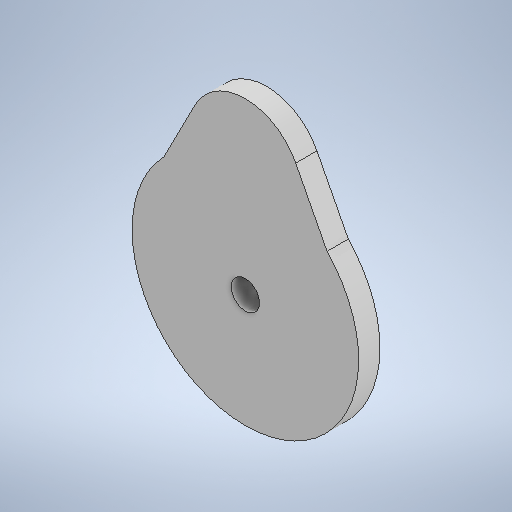
# Autodesk Inventor part: Part_Pear_Cam
Saved by Autodesk Inventor 2025 (Build 290162010, 162A)
## iProperties
Created: 2023-01-24
Part Number: Part_Pear_Cam
Material: Generic
Document SubType Name: Modeling
Designer: kani2
Density: 1 g/cm^3
Appearance: Default
Author: kani2
Autodesk Inventor part; units mm, degrees
ref_plane "YZ Plane" through (0, 0, 0) normal (1, 0, 0) x (0, 1, 0)
ref_plane "XZ Plane" through (0, 0, 0) normal (0, 1, 0) x (-1, 0, 0)
ref_plane "XY Plane" through (0, 0, 0) normal (0, 0, 1) x (1, 0, 0)
sketch "Sketch1" plane through (0, 0, 0) normal (0, 0, 1) x (1, 0, 0)
  arc A0 (-18.3123, 17.6017) -> (18.3123, 17.6017) centre (0, 0) ccw
  line L0 (-18.3123, 17.6017) -> (-11.287, 31.2218)
  line L1 (18.3123, 17.6017) -> (11.287, 31.2218)
  arc A1 (11.287, 31.2218) -> (-11.287, 31.2218) centre (0, 25.4) ccw
  dimension "d0" = 50.8
  dimension "d2" = 25.4
  constraints: 4 end point, 4 point on circle, 2 centre point, 2 tangent, 1 coincident
  measures "d0" diameter of A0
  measures "d2" distance of point (0, 0) A1.centre
extrude "Extrusion1" add sketch "Sketch1" along normal blind 4.7625
sketch "Sketch2" plane through (0, 0, 4.7625) normal (0, 0, 1) x (1, 0, 0)
  circle A0 centre (0, 0) radius 3.175
  dimension "d5" = 6.35
  constraints: 1 centre point, 1 coincident
  measures "d5" diameter of A0
extrude "Extrusion2" cut sketch "Sketch2" against normal blind 4.7625
equation "\"d0\" = d"
equation "\"d2\" = 0.5 * d"
equation "\"d\" = 50.8"
equation "\"d1\" = 0.5 * d"
body "Solid1"
